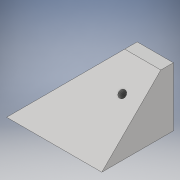
# Autodesk Inventor part: MocowanieBok2
Saved by Autodesk Inventor 2019 (Build 230136000, 136)
## iProperties
Created: 2021-12-12
Part Number: MocowanieBok2
Material: Ogólny
Document SubType Name: Modeling
Designer: Michał
Density: 1 g/cm^3
Appearance: Domyślna
Author: Michał
Autodesk Inventor part; units mm, degrees
ref_plane "YZ Plane" through (0, 0, 0) normal (1, 0, 0) x (0, 1, 0)
ref_plane "XZ Plane" through (0, 0, 0) normal (0, 1, 0) x (-1, 0, 0)
ref_plane "XY Plane" through (0, 0, 0) normal (0, 0, 1) x (1, 0, 0)
sketch "Szkic1" plane through (0, 0, 0) normal (1, 0, 0) x (0, 1, 0)
  line L0 (0, 0) -> (20, 0)
  line L1 (20, 0) -> (20, -24.25)
  line L2 (20, -24.25) -> (0, -24.25)
  line L3 (0, -24.25) -> (0, 0)
  line L4 (0, 0) -> (20, -20)
  dimension "d0" = 20
  dimension "d1" = 24.25
  dimension "d4" = 45
  constraints: 10 end point, 2 parallel, 1 horizontal, 1 perpendicular, 1 point on line
  measures "d0" distance of L0.start L0.end
  measures "d1" distance of L2.end L0.start
  measures "d4" angle of L3 L4
extrude "Wyciągnięcie proste1" add sketch "Szkic1" along normal blind 32.257 contours L4 L1 L2 L3
sketch "Szkic2" plane through (0, 0, -24.25) normal (0, 0, -1) x (-1, 0, 0)
  line L0 (0, 0) -> (0, 20) projected
  line L1 (0, 0) -> (0, 20)
  line L2 (0, 0) -> (-20, 20)
  line L3 (0, 20) -> (-32.257, 20) projected
  dimension "d5" = 45
  constraints: 4 end point, 1 point on line, 1 vertical
  measures "d5" angle of L0 L2
extrude "Wyciągnięcie proste2" cut sketch "Szkic2" against normal up to next
sketch "Szkic3" plane through (32.257, 0, -24.25) normal (0, -1, 0) x (1, 0, 0)
  line L0 (0, 24.25) -> (0, 0) projected
  line L1 (-32.257, 24.25) -> (0, 24.25) projected
  line L2 (-32.257, 24.25) -> (-32.257, 0) projected
  line L3 (-32.257, 0) -> (0, 0) projected
  point P0 (-5, 15)
  point P1 (-24.5, 7)
  dimension "d8" = 5
  dimension "d38" = 24.5
  dimension "d39" = 7
  dimension "d40" = 15
  measures "d8" distance from line of L0 point (-5, 15)
  measures "d38" distance from line of L0 point (-24.5, 7)
  measures "d39" distance from line of point (-24.5, 7) L3
  measures "d40" distance from line of L3 point (-5, 15)
hole "Otwór1" at (27.257, 0, -9.25) at (7.757, 0, -17.25) direction (0, 1, 0) diameter 2.459 depth 5 tip angle 118 thread size "M3x0.5" class "6H" standard "ISO Metric profile"
sketch "Szkic4" plane through (0, 0, 0) normal (0, 0.7071, 0.7071) x (1, 0, 0)
  line L0 (20, 28.2843) -> (32.257, 28.2843) projected
  line L1 (32.257, 28.2843) -> (32.257, 0) projected
  point P0 (0, 0)
  point P1 (25.9815, 18.6912)
  dimension "d19" = 9.5931
  dimension "d20" = 6.2755
  measures "d19" distance from line of L0 point (25.982, 18.691)
  measures "d20" distance from line of L1 point (25.982, 18.691)
hole "Otwór2" at (25.9815, 13.2167, -13.2167) direction (0, -0.7071, -0.7071) diameter 2.459 depth 5 tip angle 118 thread size "M3x0.5" class "6H" standard "ISO Metric profile"
sketch "Szkic5" plane through (0, 0, -24.25) normal (-0.7071, 0.7071, 0) x (-0.7071, -0.7071, 0)
  line L0 (0, 24.25) -> (0, 0) projected
  line L1 (0, 0) -> (-28.2843, 0) projected
  line L2 (-28.2843, 0) -> (-28.2843, 4.25) projected
  point P0 (-11.9843, 6)
  dimension "d29" = 6
  dimension "d37" = 16.3
  measures "d29" distance from line of L1 point (-11.984, 6)
  measures "d37" distance from line of L2 point (-11.984, 6)
hole "Otwór3" at (8.4742, 8.4742, -18.25) direction (0.7071, -0.7071, 0) diameter 2.459 depth 5 tip angle 118 thread size "M3x0.5" class "6H" standard "ISO Metric profile"
